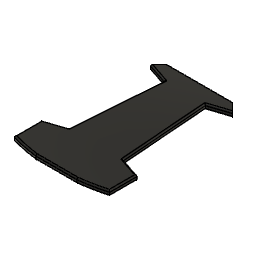
lfr1 v1 new (Autodesk Fusion 360 design; units mm, degrees)
Autodesk Fusion 360 part; units mm, degrees
sketch "Sketch1" plane through (0, 0, 0) normal (0, 0, 1) x (1, 0, 0)
  line L0 (-48.2007, 1.7996) -> (48.2007, 1.7996)
  line L1 (-48.2007, 1.7996) -> (-60.0002, -9.9999)
  line L2 (48.2007, 1.7996) -> (60.0002, -9.9999)
  line L3 (-60.0002, -9.9999) -> (-29.9999, -20)
  line L4 (60.0002, -9.9999) -> (29.9999, -20)
  line L5 (-29.9999, -20) -> (-40.001, -150.017)
  line L6 (29.9999, -20) -> (39.9997, -149.9999)
  line L7 (-40.001, -150.017) -> (-70, -160.0167)
  line L8 (-70, -160.0167) -> (-70, -200.0167)
  line L9 (39.9997, -149.9999) -> (70, -160.0001)
  line L10 (70, -160.0001) -> (70, -200.0167)
  line L11 (-30, -208.2004) -> (30, -208.2004)
  arc A0 (-70, -200.0167) -> (-30, -208.2004) centre (0, 40.2773) ccw
  arc A1 (30, -208.2004) -> (70, -200.0167) centre (0, 40.2773) ccw
  line L12 (0, 0) -> (0, -208.2004) construction
  dimension "d31" = 40
  dimension "d32" = 60
  dimension "d33" = 210
  dimension "d38" = 140
  constraint horizontal L0
  constraint perpendicular L1 L2
  constraint parallel L4 L7
  constraint vertical L8
  constraint parallel L8 L10
  constraint coincident L11.end A0
  constraint horizontal L11
  constraint concentric A0 A1
  constraint coincident L12.start origin
  constraint midpoint L11 L12.end
  constraint symmetric L1 L2 L12
  constraint symmetric L3 L4 L12
  measures "d31" distance of L7.end L8.end
  measures "d32" distance of L11.start L11.end
  measures "d33" distance of L0 L11
  measures "d38" distance of L8 L10
extrude "Extrude2" add sketch "Sketch1" along normal mid plane 7.5
fillet "Fillet1" radius 2 22 edges at (34.9998, -85, 3.75) (54.9998, -155, 3.75) (34.9998, -85, -3.75) (45.0001, -15, 3.75) (45.0001, -15, -3.75) (54.9998, -155, -3.75) (70, -180.0084, 3.75) (70, -180.0084, -3.75) (50.1672, -204.9256, 3.75) (50.1672, -204.9256, -3.75) (0, -208.2004, -3.75) (0, -208.2004, 3.75) (-50.1672, -204.9256, 3.75) (-50.1672, -204.9256, -3.75) (-70, -180.0167, 3.75) (-70, -180.0167, -3.75) (-55.0005, -155.0168, 3.75) (-55.0005, -155.0168, -3.75) (-35.0004, -85.0085, 3.75) (-35.0004, -85.0085, -3.75) (-45.0001, -15, 3.75) (-45.0001, -15, -3.75)
extrude "Extrude1" [rolled back] along distance 3.75 taper angle -60
